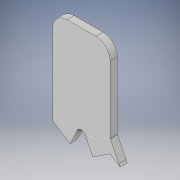
# Autodesk Inventor part: Arm_Base
Saved by Autodesk Inventor 2019 (Build 230136000, 136)
## iProperties
Created: 2019-08-29
Part Number: Arm_Base
Material: Generic
Document SubType Name: Modeling
Designer: Jorian Brusind
Density: 1 g/cm^3
Appearance: Default
Author: Jorian Brusind
Autodesk Inventor part; units mm, degrees
ref_plane "YZ Plane" through (0, 0, 0) normal (1, 0, 0) x (0, 1, 0)
ref_plane "XZ Plane" through (0, 0, 0) normal (0, 1, 0) x (-1, 0, 0)
ref_plane "XY Plane" through (0, 0, 0) normal (0, 0, 1) x (1, 0, 0)
sketch "Sketch2" plane through (0, 0, 0) normal (0, 0, 1) x (1, 0, 0)
  line L0 (0, 0) -> (100, 0)
  line L1 (100, 0) -> (100, 100)
  line L2 (100, 100) -> (0, 100)
  line L3 (0, 100) -> (0, 0)
  dimension "d24" = 100
  dimension "d25" = 100
  constraints: 8 end point, 2 parallel, 1 horizontal, 1 perpendicular
  measures "d24" distance of L2.end L1.end
  measures "d25" distance of L1.end L0.end
extrude "Extrusion3" add sketch "Sketch2" along normal blind 5
sketch "Sketch3" plane through (0, 0, 5) normal (0, 0, 1) x (1, 0, 0)
  line L0 (100, 100) -> (0, 100) projected
  line L1 (61.1065, 16.5645) -> (65.8098, 9.5096)
  ellipse E0 centre (57.8098, 14.5814) end of major axis (53.8097, 14.5816) minor radius 3.4641
  line L2 (49.8098, 9.5096) -> (54.5131, 16.5645)
  line L3 (65.8098, 9.5096) -> (77.2764, 15.2429)
  line L4 (83.9156, 31.2525) -> (78.0026, 43.0784)
  line L5 (49.8098, 26.1436) -> (54.4159, 35.3558)
  line L6 (58.3112, 37.4887) -> (58.6416, 37.4249)
  line L7 (56.9769, 37.4324) -> (57.4131, 37.502)
  line L8 (38.6658, 33.573) -> (49.8098, 26.1436)
  ellipse E1 centre (30.5481, 100.1015) end of major axis (25.0287, 91.7624) minor radius 10.0002
  line L9 (78.4473, 33.7186) -> (83.2584, 30.5112)
  line L10 (83.2584, 30.5112) -> (84.5136, 29.6744)
  line L11 (83.9156, 31.2525) -> (84.7776, 29.4984)
  line L12 (83.9156, 31.2525) -> (85.87, 31.2525) construction
  line L13 (84.7776, 29.4984) -> (84.5136, 29.6744)
  line L14 (78.4473, 33.7186) -> (77.8098, 34.1436)
  line L15 (78.4473, 33.7186) -> (79.931, 33.7186) construction
  line L16 (77.2128, 33.7456) -> (77.8098, 34.1436)
  line L17 (77.2128, 33.7456) -> (77.9303, 33.7456) construction
  line L18 (57.8098, 14.5814) -> (57.8098, 100)
  arc A0 (47.8099, 100) -> (37.8097, 90) centre (47.8099, 89.9998) ccw
  line L19 (47.8099, 89.9998) -> (57.8098, 89.9998)
  line L20 (57.8098, 89.9998) -> (67.8098, 89.9998)
  line L21 (57.8098, 89.9998) -> (67.8098, 89.9998) construction
  arc A1 (77.81, 90) -> (67.8098, 100) centre (67.8098, 89.9998) ccw
  line L22 (47.8099, 100) -> (67.8098, 100)
  line L23 (78.0026, 43.0784) -> (77.81, 43.4636)
  line L24 (78.0026, 43.0784) -> (78.4334, 43.0784) construction
  line L25 (77.81, 43.4636) -> (77.81, 43.8508)
  line L26 (65.8098, 26.1436) -> (61.2037, 35.3558)
  line L27 (37.8097, 63.9104) -> (37.8098, 35.2913)
  line L28 (38.6658, 33.573) -> (37.8098, 34.1436)
  line L29 (38.6658, 33.573) -> (39.6945, 33.573) construction
  line L30 (37.8098, 34.1436) -> (37.8098, 35.2913)
  line L31 (37.8097, 63.9104) -> (37.8097, 90)
  arc A2 (61.2037, 35.3558) -> (54.4159, 35.3558) centre (57.8098, 35.2913) ccw
  line L32 (65.8098, 26.1436) -> (77.2128, 33.7456)
  line L33 (77.81, 43.8508) -> (77.81, 90)
  line L34 (100, 0) -> (100, 100) projected
  line L35 (0, 100) -> (100, 100)
  line L36 (100, 100) -> (100, 0)
  line L37 (100, 0) -> (0, 0)
  line L38 (0, 0) -> (0, 100)
  point P0 (78.3106, 15.3544)
  point P1 (77.7245, 15.3467)
  point P2 (77.3127, 15.2462)
  point P3 (60.1591, 36.6399)
  point P4 (55.4604, 36.6398)
  point P5 (91.0098, 173.4299)
  dimension "d31" = 296.17
  dimension "d32" = 213.69
  dimension "d33" = 326.31
  dimension "d34" = 10
  dimension "d35" = 0
  dimension "d36" = 243.43
  dimension "d37" = 213.69
  constraints: 74 end point, 8 horizontal, 6 point on circle, 5 equal length, 4 vertical, 3 centre point, 3 collinear, 2 coincident, 2 parallel, 2 perpendicular, 2 point on line, 2 symmetric about line, 8 other
  measures "d34" distance of L19.end L20.end
  measures "d35" distance between parallel lines of L20 L21
extrude "Extrusion4" cut sketch "Sketch3" against normal blind 10 contours L34 L37 L38 L0 E1 A0 L31 L27 L30 L28 L8 L5 A2 L26 L32 L16 L14 L9 L10 L13 L11 L4 L23 L25 L33 A1 | A0 E1 L0 | E1 L0 | E0 picked at (31.1987, 94.7741)
body "Solid3"
